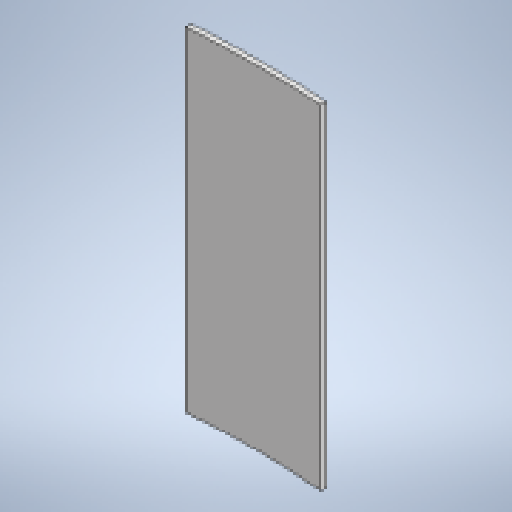
# Autodesk Inventor part: ДМФ 01 13 Барабан усилитель v2.0
Saved by Autodesk Inventor 2025.3 (Build 293356030, 356C)
## iProperties
Created: 2024-04-30
Part Number: ДМФ 01 13 Барабан усилитель v2.0
Material: Generic
Document SubType Name: Sheet Metal
Designer: pokla
Stock Number: Барабан_Сектор_Усилителя
Density: 1 g/cm^3
Sheet Metal Rule: Default
Sheet Metal Width: 0,000 mm
Sheet Metal Length: 0,000 mm
Sheet Metal Area: 0,000 mm^2
Appearance: Default
Author: pokla
Autodesk Inventor part; units mm, degrees
ref_plane "YZ Plane" through (0, 0, 0) normal (1, 0, 0) x (0, 1, 0)
ref_plane "XZ Plane" through (0, 0, 0) normal (0, 1, 0) x (-1, 0, 0)
ref_plane "XY Plane" through (0, 0, 0) normal (0, 0, 1) x (1, 0, 0)
sketch "Sketch1" plane through (0, 0, 0) normal (0, 0, 1) x (1, 0, 0)
  circle A0 centre (0, 0) radius 242
  line L0 (-25, 364.1428) -> (25, 364.1428)
  line L1 (25, 364.1428) -> (25, 240.7052)
  line L2 (25, 240.7052) -> (-25, 240.7052)
  line L3 (-25, 240.7052) -> (-25, 364.1428)
  circle A1 centre (0, 0) radius 365
  dimension "d28" = 730
  dimension "d26" = 484
  dimension "d27" = 50
  measures "d26" diameter of A0
  measures "d27" distance of L1.end L2.end
extrude "Plate1" add sketch "Sketch1" against normal blind 2 contours A0 L3 L0 L1 | L0 A1
equation "\"d26\" = Колесо_диам_3 + 2 * Thickness"
equation "\"d15\" = Thickness"
equation "\"BendRadius\" = Thickness"
equation "\"BendReliefWidth\" = Thickness"
equation "\"BendReliefDepth\" = 0.5 * Thickness"
equation "\"CornerReliefSize\" = 4 * Thickness"
equation "\"MinimumRemnant\" = 2 * Thickness"
equation "\"TransitionRadius\" = BendRadius"
equation "\"JacobiRadiusSize\" = BendRadius"
equation "\"GapSize\" = Thickness"
equation "\"Колесо_диам_3\" = 480"
equation "\"Thickness\" = 2"
body "Solid1"
